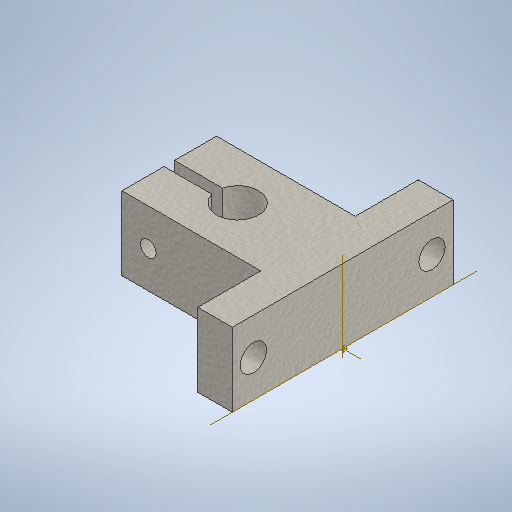
# Autodesk Inventor part: Shaft support - Stock
Saved by Autodesk Inventor 2025.2 (Build 292293000, 293)
## iProperties
Created: 2025-01-25
Part Number: Shaft support - Stock
Material: Generic
Document SubType Name: Modeling
Designer: caomi
Density: 1 g/cm^3
Appearance: Default
Author: caomi
Autodesk Inventor part; units mm, degrees
ref_plane "YZ Plane" through (0, 0, 0) normal (1, 0, 0) x (0, 1, 0)
ref_plane "XZ Plane" through (0, 0, 0) normal (0, 1, 0) x (-1, 0, 0)
ref_plane "XY Plane" through (0, 0, 0) normal (0, 0, 1) x (1, 0, 0)
sketch "Sketch1" plane through (0, 0, 0) normal (0, 1, 0) x (-1, 0, 0)
  line L0 (16, 0) -> (0, 0)
  line L1 (0, 0) -> (0, -21)
  line L2 (0, -21) -> (6.6, -21)
  line L3 (6.6, -21) -> (6.6, -9)
  line L4 (6.6, -9) -> (33, -9)
  line L5 (33, -9) -> (33, -1)
  circle A0 centre (20, 0) radius 4
  line L6 (23.873, -1) -> (33, -1)
  line L7 (0, 0) -> (0, 21)
  line L8 (0, 21) -> (6.6, 21)
  line L9 (6.6, 21) -> (6.6, 9)
  line L10 (6.6, 9) -> (33, 9)
  line L11 (33, 9) -> (33, 1)
  circle A1 centre (20, 0) radius 4
  line L12 (23.873, 1) -> (33, 1)
  dimension "d0" = 6.6
  dimension "d1" = 21
  dimension "d2" = 1
  dimension "d3" = 9
  dimension "d4" = 8
  dimension "d5" = 33
  dimension "d19" = 20
  constraints: 26 end point, 6 symmetric about line, 5 perpendicular, 3 point on line, 2 horizontal, 2 point on circle, 1 centre point, 1 line through centre, 3 other
  measures "d0" distance of L1.end L2.end
  measures "d1" distance of L0.end L1.end
  measures "d2" distance between parallel lines of L6 L0
  measures "d3" distance between parallel lines of L4 L0
  measures "d4" diameter of A0
  measures "d5" distance between parallel lines of L1 L5
  measures "d19" distance from line of A0.centre L1
extrude "Extrusion1" add sketch "Sketch1" along normal blind 14 contours A0 L6 L5 L4 L3 L2 L1 L0 | L0 L7 L8 L9 L10 L11 L12 A0
sketch "Sketch2" plane through (0, 0, 21) normal (1, 0, 0) x (0, 0, -1)
  circle A0 centre (38, 7) radius 2.5
  line L0 (21, 26.3461) -> (21, -5.4737) construction
  line L1 (0, 14) -> (42, 14) projected
  line L2 (42, 0) -> (42, 14) projected
  circle A1 centre (4, 7) radius 2.5
  point P0 (21, 0)
  point P1 (21, 14)
  point P2 (42, 7)
  dimension "d10" = 5
  dimension "d14" = 4
  constraints: 2 centre point, 2 end point, 2 midpoint, 1 horizontal alignment, 1 point on line, 1 symmetric about line, 1 vertical, 1 other
  measures "d10" diameter of A0
  measures "d14" distance from line of A0.centre L2
extrude "Extrusion2" cut sketch "Sketch2" against normal blind 14
sketch "Sketch3" plane through (-6.6, 0, -9) normal (0, 0, -1) x (-1, 0, 0)
  circle A0 centre (21.4, 7) radius 1.5
  line L0 (26.4, 0) -> (26.4, 14) projected
  point P0 (-6.6, 0)
  point P1 (26.4, 7)
  dimension "d15" = 3
  dimension "d16" = 5
  constraints: 1 centre point, 1 horizontal alignment, 1 midpoint
  measures "d15" diameter of A0
  measures "d16" distance from line of A0.centre L0
extrude "Extrusion3" cut sketch "Sketch3" against normal up to surface (18 mm away)
equation "\"d17\" = d15"
body "Solid1"
